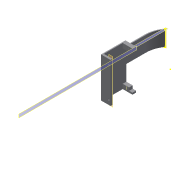
# Autodesk Inventor part: CollectorChute25DegreesRoof
Saved by Autodesk Inventor 2018 (Build 220112000, 112)
## iProperties
Created: 2019-01-27
Part Number: CollectorChute25DegreesRoof
Material: Generic
Document SubType Name: Modeling
Designer: ball
Density: 1 g/cm^3
Appearance: Default
Author: ball
Autodesk Inventor part; units mm, degrees
ref_plane "YZ Plane" through (0, 0, 0) normal (1, 0, 0) x (0, 1, 0)
ref_plane "XZ Plane" through (0, 0, 0) normal (0, 1, 0) x (-1, 0, 0)
ref_plane "XY Plane" through (0, 0, 0) normal (0, 0, 1) x (1, 0, 0)
ref_plane "Work Plane1" through (0, 0, 0) normal (0, 0, 1) x (1, 0, 0)
sketch "Sketch1" plane through (0, 0, 0) normal (0, 0, 1) x (1, 0, 0)
  line L0 (-2.5, -8) -> (-12, -8) construction
  line L1 (-2.5, 96) -> (-2.5, -8) construction
  line L2 (-12, 96) -> (-12, -8) construction
  line L3 (-2.5, 96) -> (-12, 96) construction
  line L4 (-27.9, -8) -> (-27.9, 96)
  line L5 (-3.175, 96) -> (-3.175, -8)
  line L6 (-27.9, -8) -> (-3.175, -8)
  line L7 (-27.9, 96) -> (-3.175, 96)
  circle A0 centre (-8, 4) radius 2 construction
  circle A1 centre (-8, 84) radius 2 construction
  circle A2 centre (-8, 4) radius 2.2479
  circle A3 centre (-8, 84) radius 2.2479
  point P0 (0, 0)
  dimension "d1" = 0.675
  dimension "d2" = 4.4958
  dimension "d3" = 4.4958
  dimension "d7" = 25.4
  constraints: 16 end point, 4 centre point, 4 point on line, 3 horizontal, 2 coincident, 2 vertical, 1 collinear, 8 other
  measures "d1" distance between parallel lines of L1 L5
  measures "d2" diameter of A2
  measures "d3" diameter of A3
  measures "d7" distance between parallel lines of L4 L1
extrude "Extrusion1" add sketch "Sketch1" along normal blind 5.08
sketch "Sketch2" plane through (0, 0, 0) normal (0, 0, -1) x (-1, 0, 0)
  line L0 (3.175, 96) -> (27.9, 96) projected
  line L1 (27.9, -8) -> (3.175, -8) projected
  line L2 (27.9, 96) -> (25.36, 96)
  line L3 (25.36, 96) -> (25.36, -8)
  line L4 (25.36, -8) -> (27.9, -8)
  line L5 (27.9, -8) -> (27.9, 96)
  line L6 (-64, -1.0267) -> (8, -1.0267) construction
  point P0 (0, 0)
  dimension "d6" = 2.54
  constraints: 10 end point, 2 horizontal, 2 parallel, 1 perpendicular, 1 point on line, 2 other
  measures "d6" distance of L4.end L3.end
ref_plane "Work Plane3" through (0, 92, -38.5) normal (-1, 0, 0) x (0, 0, 1)
sketch "Sketch3" plane through (0, 92, -38.5) normal (-1, 0, 0) x (0, 0, 1)
  line L0 (-8, 4) -> (-10.5, 4) construction
  line L1 (-10.5, -5.5) -> (-10.5, 4) construction
  line L2 (-20, -0.42) -> (-10.5, -0.42)
  line L3 (-20, -0.42) -> (-20, -90.5) construction
  line L4 (-10.5, 4) -> (-20, 4)
  line L5 (-20, 4) -> (-20, -0.42)
  line L6 (-20, -0.42) -> (-10.5, -0.42)
  line L7 (-10.5, -0.42) -> (-10.5, 4)
  line L8 (-20, -95.58) -> (-10.5, -95.58) construction
  line L9 (-10.5, -95.58) -> (-10.5, -90.5) construction
  line L10 (-20, -0.42) -> (-20, -90.5) construction
  line L11 (-8, -100) -> (-10.5, -100) construction
  line L12 (-10.5, -95.58) -> (-20, -95.58)
  line L13 (-20, -95.58) -> (-20, -100)
  line L14 (-20, -100) -> (-10.5, -100)
  line L15 (-10.5, -100) -> (-10.5, -95.58)
  point P0 (38.5, -92)
  constraints: 32 end point, 6 horizontal, 4 parallel, 4 vertical, 2 perpendicular, 11 other
extrude "Extrusion2" add sketch "Sketch3" along normal blind 25.4
ref_plane "Work Plane4" through (-16.011, -1.04, -53.75) normal (-1, 0, 0) x (0, 0, 1)
sketch "Sketch4" plane through (0, 91.58, -58.5) normal (0, -1, 0) x (1, 0, 0)
  line L0 (-7.9375, 9.525) -> (-7.9375, 0) construction
  line L1 (0, 0) -> (-25.4, 0) construction
  line L2 (-8.5725, 9.525) -> (-8.5725, 0) construction
  line L3 (-25.4, 0) -> (-25.4, 9.5) projected
  line L4 (-8.5725, 9.525) -> (-25.4, 9.525)
  line L5 (-25.4, 9.525) -> (-25.4, 0)
  line L6 (-25.4, 0) -> (-8.5725, 0)
  line L7 (-8.5725, 0) -> (-8.5725, 9.525)
  point P0 (0, 58.5)
  dimension "d10" = 0.635
  constraints: 12 end point, 3 parallel, 1 horizontal, 1 perpendicular, 1 point on line, 1 vertical
  measures "d10" distance between parallel lines of L0 L2
ref_plane "Work Plane5" through (-16.5193, 84.005, -147.6492) normal (0, -1, 0) x (1, 0, 0)
extrude "Extrusion3" add sketch "Sketch4" along normal up to surface (7.575 mm away)
sketch "Sketch5" plane through (0, -3.58, -49) normal (0, 1, 0) x (1, 0, 0)
  line L0 (-8, 0) -> (-8, 9.5) construction
  line L1 (-8.635, 0) -> (-8.635, 9.5) construction
  line L2 (0, 9.5) -> (-25.4, 9.5) construction
  line L3 (-8.635, 0) -> (-25.4, 0) construction
  line L4 (-25.4, 0) -> (-25.4, 9.5) construction
  line L5 (-25.4, 9.5) -> (-8.635, 9.5) construction
  line L6 (-8.635, 9.5) -> (-8.635, 0) construction
  line L7 (0, 9.5) -> (-25.4, 9.5) projected
  line L8 (-8.635, 0) -> (-25.4, 0)
  line L9 (-25.4, 0) -> (-25.4, 9.5)
  line L10 (-25.4, 9.5) -> (-8.635, 9.5)
  line L11 (-8.635, 9.5) -> (-8.635, 0)
  point P0 (0, -49)
  dimension "d13" = 0.635
  constraints: 20 end point, 5 parallel, 2 horizontal, 2 perpendicular, 1 vertical, 2 other
  measures "d13" distance between parallel lines of L0 L1
ref_plane "Work Plane6" through (-16.214, 3.995, -107.6746) normal (0, 1, 0) x (0, 0, 1)
extrude "Extrusion4" add sketch "Sketch5" along normal up to surface (7.575 mm away)
extrude "Extrusion5" add sketch "Sketch2" along normal up to surface (58.5 mm away)
ref_plane "Work Plane7" through (-16, 84.005, -58.5129) normal (0, -1, 0) x (0, 0, 1)
ref_plane "Work Plane8" through (-15.9869, 84.005, -147.6244) normal (-0.0001466, 0, 1) x (0, 1, 0)
sketch "Sketch7" plane through (-15.9869, 84.005, -147.6244) normal (-0.0001466, 0, 1) x (0, 1, 0)
  spline S0 degree 3 poles (-40.0045, -2.04) (-26.4732, -3.101) (-13.8537, -3.2752) (0, -2.9022) knots -4.216778 -4.216778 -4.216778 -4.216778 -0.050074 -0.050074 -0.050074 -0.050074 projected
  point P0 (-84.005, -16.0086)
ref_plane "Work Plane11" through (-9.0939, 44, -144.0149) normal (0, -1, 0) x (1, 0, -0.0000527)
sketch "Sketch8" plane through (-16, 84.005, -58.5129) normal (0, -1, 0) x (0, 0, 1)
  line L0 (0.0129, -16) -> (0.0129, 11.9) projected
  line L1 (0.0129, 11.9) -> (-49.1107, 11.9)
  line L2 (-49.1107, 9.36) -> (0.0129, 9.36)
  line L3 (0.0129, 9.36) -> (0.0129, 11.9)
  spline S0 degree 3 poles (-89.1111, -2.9152) (-81.5412, -1.4973) (-73.7884, -0.8377) (-66.09, -0.5489) knots -2.311143 -2.311143 -2.311143 -2.311143 0 0 0 0 construction
  line L4 (-89.1111, -2.9152) -> (-89.1111, -0.3752)
  line L5 (-49.1107, 11.9) -> (-49.1107, 9.36)
  point P0 (58.5129, -16)
  dimension "d22" = 2.54
  dimension "d23" = 2.54
  dimension "d30" = 49.1236
  constraints: 10 end point, 2 vertical, 1 horizontal, 1 parallel
  measures "d22" distance of L2.start L1.end
  measures "d23" distance of L4.start L4.end
  measures "d30" distance between parallel lines of L5 L3
extrude "Extrusion6" add sketch "Sketch8" along normal up to surface (40.005 mm away)
ref_plane "Work Plane9" through (-15.9871, 84.005, -146.3544) normal (-0.0001466, 0, 1) x (0, 1, 0)
sketch "Sketch11" plane through (-15.9871, 84.005, -146.3544) normal (-0.0001466, 0, 1) x (0, 1, 0)
  spline S0 degree 3 poles (0, -5.4882) (-13.8521, -5.8632) (-26.4769, -5.6797) (-40.0045, -4.616) knots -4.128271 -4.128271 -4.128271 -4.128271 -0.050202 -0.050202 -0.050202 -0.050202 construction
  line L0 (0, -5.4882) -> (0, -2.9022) construction
  spline S1 degree 3 poles (-40.0045, -2.04) (-26.4732, -3.101) (-13.8537, -3.2752) (0, -2.9022) knots -4.216778 -4.216778 -4.216778 -4.216778 -0.050074 -0.050074 -0.050074 -0.050074 construction
  line L1 (-40.0045, -4.616) -> (-40.0045, -2.04) construction
  point P0 (-84.005, -16.0086)
sketch "Sketch12" plane through (-16, 84.005, -58.5129) normal (0, -1, 0) x (0, 0, 1)
  line L0 (-87.8408, -4.6289) -> (-87.8412, -2.0529) construction
  line L1 (-49.1107, 11.9) -> (-49.1107, 9.36) projected
  line L2 (-49.1107, 11.9) -> (-49.1107, 9.36)
  arc A0 (-49.1107, 11.9) -> (-87.8412, -2.0529) centre (-43.4658, -64.4998) ccw
  arc A1 (-49.1107, 9.36) -> (-87.8408, -4.6289) centre (-43.4095, -67.034) ccw
  line L3 (-87.8412, -2.0529) -> (-87.8408, -4.6289)
  point P0 (58.5129, -16)
  dimension "d32" = 76.6064
  constraints: 4 end point, 4 point on circle, 2 centre point, 2 collinear
  measures "d32" radius of A1
ref_plane "Work Plane10" through (-9.0939, 44, -144.0149) normal (0, -1, 0) x (1, 0, -0.0000527)
extrude "Extrusion8" add sketch "Sketch12" along normal up to surface (40.005 mm away)
sketch "Sketch13" plane through (-27.9, 44, -107.6236) normal (0, -1, 0) x (1, 0, 0)
  line L0 (16.5289, -38.7301) -> (13.9529, -38.7305) projected
  arc A0 (2.54, 0) -> (16.5289, -38.7301) centre (78.934, 5.7012) ccw projected
  arc A1 (0, 0) -> (13.9529, -38.7305) centre (76.3998, 5.6449) ccw projected
  line L1 (0, 49.1236) -> (2.54, 49.1236) projected
  line L2 (0, 0) -> (0, 49.1236) projected
  line L3 (2.54, 49.1236) -> (2.54, 0) projected
  line L4 (2.54, 49.1236) -> (2.54, 0) projected
  line L5 (0, 0) -> (2.54, 0)
  point P0 (27.9, 107.6236)
  constraints: 2 end point, 1 horizontal
revolve "Revolution1" add sketch "Sketch13" angle 90 about axis through (-27.9, 44, -107.6236) along (-1, 0, 0) contours L0 A1 L5 A0
sketch "Sketch14" plane through (0, -8, -58.5) normal (0, 0, -1) x (-1, 0, 0)
  line L0 (25.36, 11.995) -> (25.36, 52) projected
  line L1 (27.9, 52) -> (25.36, 52)
  line L2 (25.36, 52) -> (25.36, 11.995)
  line L3 (27.9, 11.995) -> (27.9, 52)
  line L4 (25.36, 11.995) -> (8.635, 11.995) construction
  line L5 (0, 0) -> (27.9, 0) construction
  line L6 (11.3711, 13.2699) -> (11.3711, 52) construction
  line L7 (16.011, 9.5) -> (16.011, 4.42) construction
  line L8 (16.011, 11.995) -> (16.011, 0) construction
  line L9 (8.635, 11.995) -> (25.36, 11.995) projected
  line L10 (25.36, 11.995) -> (27.9, 11.995)
  point P0 (0, 8)
  point P1 (17.281, 11.995)
  constraints: 10 end point, 2 point on line, 1 collinear, 1 horizontal, 1 parallel, 1 perpendicular
sketch "Sketch15" plane through (-27.9, 44, -107.6236) normal (0, 0, 1) x (1, 0, 0)
  line L0 (13.9529, -38.7305) -> (16.5289, -38.7301) projected
  arc A0 (2.54, 0) -> (16.5289, -38.7301) centre (78.934, 5.7012) ccw projected
  line L1 (0, 0) -> (2.54, 0) projected
  arc A1 (0, 0) -> (13.9529, -38.7305) centre (76.3998, 5.6449) ccw projected
  point P0 (27.9, -44)
loft "Loft2" add profiles "Sketch14" section 2 edges at (-12.6591, 5.2697, -107.6236) (-21.0167, 23.6774, -107.6236) (-26.63, 44, -107.6236) (-23.5739, 23.68, -107.6236)
body "Solid1"
